Cam Halter 2 (Autodesk Fusion 360 design; units mm, degrees)
Autodesk Fusion 360 part; units mm, degrees
sketch "Sketch1" plane through (0, 0, 0) normal (0, 0, 1) x (1, 0, 0)
  line L0 (0, 0) -> (40, 0)
  line L1 (40, 0) -> (40, 15)
  line L2 (40, 15) -> (0, 15)
  line L3 (0, 15) -> (0, 0)
  circle A0 centre (6, 7.5) radius 1.25
  circle A1 centre (34, 7.5) radius 1.25
  line L4 (0, 7.5) -> (40, 7.5)
  point P0 (0, 7.5)
  point P1 (40, 7.5)
  dimension "d1" = 40
  dimension "d2" = 15
  dimension "d3" = 2.5
  dimension "d4" = 2.5
  dimension "d5" = 6
  dimension "d6" = 6
  constraint horizontal L0
  constraint vertical L1
  constraint horizontal L2
  constraint vertical L3
  constraint coincident L0.start L3.end
  constraint midpoint L3 P0
  constraint midpoint L1 P1
  constraint coincident P0 L4.start
  constraint coincident P1 L4.end
  constraint coincident A0.centre L4
  constraint coincident A1.centre L4
  measures "d1" distance of L0.start L0.end
  measures "d2" distance of L0.start L2.end
  measures "d3" diameter of A0
  measures "d4" diameter of A1
  measures "d5" horizontal distance of A0.centre P0
  measures "d6" distance of L1 A1.centre
extrude "Extrude1" add sketch "Sketch1" along normal blind 1.5 contours L0 L1 L3 A0 A1 L4 | L1 L2 L3 A0 A1 L4
sketch "Sketch2" plane through (0, 0, 0) normal (0, -1, 0) x (1, 0, 0)
  line L0 (0, 0) -> (40, 0)
  line L1 (40, 0) -> (40, 1.5)
  line L2 (40, 1.5) -> (0, 1.5)
  line L3 (0, 1.5) -> (0, 0)
  circle A0 through (23.5, 6.5, 0) (18.25, 9.3483, 1.0367) (18.25, 3.6517, -1.0367)
  circle A1 through (25, 6.5, 0) (17.5, 10.569, 1.481) (17.5, 2.431, -1.481)
  point P0 (20, 1.5)
  dimension "d9" = 7
  dimension "d10" = 10
  dimension "d15" = 5
  constraint midpoint L2 P0
extrude "Extrude4" add sketch "Sketch2" along normal blind 2 contours A0 | A1 in plane through (0, 2.0891, 0.7604) normal (0, -0.939693, -0.34202)
extrude "Extrude5" add sketch "Sketch2" against normal blind 10 contours A1 in plane through (0, 2.0891, 0.7604) normal (0, -0.939693, -0.34202)
sketch "Sketch3" plane through (0, 0, 1.5) normal (0, 0, 1) x (-1, 0, 0)
  ellipse E0 centre (-20, 13.7374) end of major axis (-20, 28.3564) minor radius 5 (-21.7101, 0) -> (-18.2899, 0) ccw
  line L0 (-21.7101, 0) -> (-40, 0)
  line L1 (-40, 0) -> (-40, -15)
  line L2 (-40, -15) -> (0, -15)
  line L3 (0, -15) -> (0, 0)
  line L4 (0, 0) -> (-18.2899, 0)
  circle A0 centre (-6, -7.5) radius 1.25
  circle A1 centre (-34, -7.5) radius 1.25
  line L5 (-24.5031, 0) -> (-15.5211, 0)
  line L6 (-15.5211, 0) -> (-15.5211, -11.2767)
  line L7 (-15.5211, -11.2767) -> (-24.5031, -11.2767)
  line L8 (-24.5031, -11.2767) -> (-24.5031, 0)
  point P0 (-24.5031, 0)
  constraint horizontal L5
  constraint vertical L6
  constraint horizontal L7
  constraint vertical L8
  constraint coincident P0 L5.start
extrude "Extrude6" add sketch "Sketch3" along normal blind 4 contours E0 L0 L4 L5 L6 L7 L8
extrude "Extrude7" cut sketch "Sketch2" against normal blind 15 contours A0 in plane through (0, 2.0891, 0.7604) normal (0, -0.939693, -0.34202)
